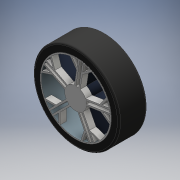
# Autodesk Inventor part: rueda
Saved by Autodesk Inventor 2016 (Build 200138000, 138)
## iProperties
Created: 2017-12-28
Part Number: rueda
Material: Genérico
Document SubType Name: Sheet Metal
Designer: David
Density: 1 g/cm^3
Sheet Metal Rule: Por defecto_mm
Appearance: Valor por defecto
Author: David
Autodesk Inventor part; units mm, degrees
ref_plane "YZ Plane" through (0, 0, 0) normal (1, 0, 0) x (0, 1, 0)
ref_plane "XZ Plane" through (0, 0, 0) normal (0, 1, 0) x (-1, 0, 0)
ref_plane "XY Plane" through (0, 0, 0) normal (0, 0, 1) x (1, 0, 0)
sketch "Boceto1" plane through (0, 0, 0) normal (0, 1, 0) x (-1, 0, 0)
  line L0 (0, 0) -> (10.773409, 0) construction
  line L1 (0, 0) -> (5.876404, 0) construction
  line L2 (0, 0) -> (5.876414, 0) construction
  line L3 (2.696241, -2.108582) -> (2.892291, -2.304632)
  line L4 (2.092671, -2.708608) -> (2.372911, -2.990503)
  line L5 (2.372911, -2.990503) -> (7.29151, -7.938146)
  line L6 (1.666633, -2.989677) -> (4.8298, -6.171522)
  line L7 (4.8298, -6.171522) -> (4.8298, -9.636042)
  line L8 (5.341204, -9.362255) -> (5.341204, -6.665792)
  line L9 (5.341204, -6.665792) -> (6.925478, -8.259421)
  line L10 (2.694469, -2.10681) -> (2.976364, -2.38705)
  line L11 (2.976364, -2.38705) -> (7.924007, -7.305649)
  line L12 (2.975538, -1.680772) -> (6.157383, -4.843939)
  line L13 (6.157383, -4.843939) -> (9.621903, -4.843939)
  line L14 (9.348116, -5.355343) -> (6.651653, -5.355343)
  line L15 (6.651653, -5.355343) -> (8.245282, -6.939617)
  line L16 (7.923737, -7.305381) -> (7.924595, -7.306234)
  line L17 (8.244685, -6.939024) -> (8.246514, -6.940842)
  line L18 (9.347907, -5.355343) -> (9.354174, -5.355343)
  line L19 (9.62164, -4.843939) -> (9.628942, -4.843939)
  line L20 (7.148707, 4.671206) -> (9.1479, 5.697269)
  line L21 (7.98196, 7.235695) -> (7.148707, 4.671206)
  line L22 (6.509596, 4.35916) -> (7.580192, 7.654114)
  line L23 (2.518001, 2.310518) -> (6.509596, 4.35916)
  line L24 (3.189966, 2.093051) -> (9.396738, 5.278608)
  line L25 (3.577407, 1.332656) -> (9.802826, 4.481616)
  line L26 (2.836332, 1.911553) -> (3.189966, 2.093051)
  line L27 (3.222711, 1.153243) -> (3.577407, 1.332656)
  line L28 (3.358369, 0.661201) -> (7.361957, 2.686308)
  line L29 (7.990067, 3.019944) -> (9.995266, 4.03422)
  line L30 (10.554556, 2.186691) -> (7.990067, 3.019944)
  line L31 (7.361957, 2.686308) -> (10.656911, 1.615712)
  line L32 (-2.233509, 8.242307) -> (-2.591569, 10.460723)
  line L33 (-4.414993, 9.827248) -> (-2.233509, 8.242307)
  line L34 (-2.134232, 7.538048) -> (-4.937087, 9.574442)
  line L35 (-1.419328, 3.10875) -> (-2.134232, 7.538048)
  line L36 (-1.004856, 3.680627) -> (-2.116503, 10.568008)
  line L37 (-0.161952, 3.81413) -> (-1.233031, 10.707937)
  line L38 (-0.94152, 3.288215) -> (-1.004856, 3.680627)
  line L39 (-0.100927, 3.421351) -> (-0.161952, 3.81413)
  line L40 (0.408954, 3.398321) -> (-0.279861, 7.831752)
  line L41 (-0.403071, 8.53222) -> (-0.748064, 10.752705)
  line L42 (1.181871, 10.713704) -> (-0.403071, 8.53222)
  line L43 (-0.279861, 7.831752) -> (1.756533, 10.634607)
  line L44 (-8.529092, 0.42282) -> (-10.749577, 0.767813)
  line L45 (-10.710576, -1.162121) -> (-8.529092, 0.42282)
  line L46 (-7.828624, 0.29961) -> (-10.631479, -1.736783)
  line L47 (-3.395193, -0.389204) -> (-7.828624, 0.29961)
  line L48 (-3.811002, 0.181701) -> (-10.704809, 1.25278)
  line L49 (-3.677499, 1.024606) -> (-10.56488, 2.136253)
  line L50 (-3.418223, 0.120676) -> (-3.811002, 0.181701)
  line L51 (-3.285087, 0.961269) -> (-3.677499, 1.024606)
  line L52 (-3.105622, 1.439077) -> (-7.53492, 2.153981)
  line L53 (-8.239179, 2.253258) -> (-10.457595, 2.611318)
  line L54 (-9.82412, 4.434742) -> (-8.239179, 2.253258)
  line L55 (-7.53492, 2.153981) -> (-9.571314, 4.956836)
  line L56 (-3.03776, -7.98099) -> (-4.052036, -9.986188)
  line L57 (-2.204507, -10.545478) -> (-3.03776, -7.98099)
  line L58 (-2.704124, -7.352879) -> (-1.633529, -10.647833)
  line L59 (-0.679017, -3.349292) -> (-2.704124, -7.352879)
  line L60 (-1.350472, -3.568329) -> (-4.499432, -9.793748)
  line L61 (-2.110867, -3.180889) -> (-5.296425, -9.38766)
  line L62 (-1.171059, -3.213633) -> (-1.350472, -3.568329)
  line L63 (-1.929369, -2.827255) -> (-2.110867, -3.180889)
  line L64 (-2.328334, -2.508923) -> (-4.376976, -6.500518)
  line L65 (-4.689022, -7.13963) -> (-5.715085, -9.138822)
  line L66 (-7.253511, -7.972883) -> (-4.689022, -7.13963)
  line L67 (-4.376976, -6.500518) -> (-7.67193, -7.571114)
  arc A0 (3.222711, 1.153243) -> (2.83856, 1.912696) centre (0, 0) ccw
  arc A1 (2.979517, -1.684728) -> (3.358369, 0.661201) centre (0, 0) ccw
  arc A2 (2.092671, -2.708608) -> (2.696245, -2.108576) centre (0, 0) ccw
  arc A3 (-0.68155, -3.354299) -> (1.666633, -2.989677) centre (0, 0) ccw
  arc A4 (2.522993, 2.31308) -> (0.408954, 3.398321) centre (0, 0) ccw
  arc A5 (-0.100927, 3.421351) -> (-0.941919, 3.290687) centre (0, 0) ccw
  arc A6 (-1.420222, 3.11429) -> (-3.105622, 1.439077) centre (0, 0) ccw
  arc A7 (-3.285087, 0.961269) -> (-3.420698, 0.12106) centre (0, 0) ccw
  arc A8 (-3.400738, -0.388343) -> (-2.328334, -2.508923) centre (0, 0) ccw
  arc A9 (-1.929369, -2.827255) -> (-1.172189, -3.215868) centre (0, 0) ccw
  line L68 (-2.205227, -10.543261) -> (-2.202798, -10.551206)
  line L69 (-1.634443, -10.645018) -> (-1.631353, -10.654528)
  line L70 (-4.051656, -9.985437) -> (-4.05282, -9.987739)
  line L71 (-4.499261, -9.793408) -> (-4.499807, -9.794489)
  line L72 (-10.619132, -1.727812) -> (-10.637174, -1.740921)
  line L73 (-10.708499, -1.160612) -> (-10.715477, -1.165682)
  line L74 (-10.747959, 0.767562) -> (-10.751294, 0.76808)
  line L75 (-10.702047, 1.252351) -> (-10.705629, 1.252907)
  line L76 (-4.936194, 9.573793) -> (-4.942782, 9.578579)
  line L77 (-4.413036, 9.825826) -> (-4.419894, 9.830809)
  line L78 (-2.591187, 10.458357) -> (-2.591845, 10.462438)
  line L79 (-2.116332, 10.56695) -> (-2.116636, 10.568828)
  line L80 (7.5795, 7.651986) -> (7.582367, 7.660809)
  line L81 (7.981253, 7.233517) -> (7.983833, 7.241456)
  line L82 (9.145324, 5.695947) -> (9.149446, 5.698063)
  line L83 (9.394975, 5.277704) -> (9.397476, 5.278988)
  circle A10 centre (0, 0) radius 11.15
  arc A11 (9.149446, 5.698063) -> (7.983833, 7.241456) centre (0, 0) ccw
  arc A12 (9.802826, 4.481616) -> (9.397476, 5.278988) centre (0, 0) ccw
  arc A13 (10.554556, 2.186691) -> (9.995266, 4.03422) centre (0, 0) ccw
  arc A14 (9.628942, -4.843939) -> (10.656911, 1.615712) centre (0, 0) ccw
  arc A15 (8.246514, -6.940842) -> (9.354174, -5.355343) centre (0, 0) ccw
  arc A16 (7.29151, -7.938146) -> (7.924595, -7.306234) centre (0, 0) ccw
  arc A17 (5.341204, -9.362255) -> (6.925478, -8.259421) centre (0, 0) ccw
  arc A18 (-5.296425, -9.38766) -> (-4.499807, -9.794489) centre (0, 0) ccw
  arc A19 (-4.05282, -9.987739) -> (-2.202798, -10.551206) centre (0, 0) ccw
  arc A20 (-1.631353, -10.654528) -> (4.8298, -9.636042) centre (0, 0) ccw
  arc A21 (-7.253511, -7.972883) -> (-5.715085, -9.138822) centre (0, 0) ccw
  arc A22 (7.582367, 7.660809) -> (1.756533, 10.634607) centre (0, 0) ccw
  arc A23 (1.181871, 10.713704) -> (-0.748064, 10.752705) centre (0, 0) ccw
  arc A24 (-1.233031, 10.707937) -> (-2.116636, 10.568828) centre (0, 0) ccw
  arc A25 (-2.591845, 10.462438) -> (-4.419894, 9.830809) centre (0, 0) ccw
  arc A26 (-4.942782, 9.578579) -> (-9.571314, 4.956836) centre (0, 0) ccw
  arc A27 (-9.82412, 4.434742) -> (-10.457595, 2.611318) centre (0, 0) ccw
  arc A28 (-10.56488, 2.136253) -> (-10.705629, 1.252907) centre (0, 0) ccw
  arc A29 (-10.751294, 0.76808) -> (-10.715477, -1.165682) centre (0, 0) ccw
  arc A30 (-10.637174, -1.740921) -> (-7.67193, -7.571114) centre (0, 0) ccw
  point P0 (9.147151, 5.696885)
  point P1 (7.981896, 7.235496)
  point P2 (7.58011, 7.653864)
  point P3 (9.396399, 5.278435)
  point P4 (-2.591434, 10.459892)
  point P5 (-4.414824, 9.827125)
  point P6 (-4.936874, 9.574287)
  point P7 (-2.116443, 10.567633)
  point P8 (-10.748746, 0.767684)
  point P9 (-10.710407, -1.161998)
  point P10 (-10.631266, -1.736629)
  point P11 (-10.704433, 1.252722)
  point P12 (-2.204572, -10.54528)
  point P13 (-1.63361, -10.647583)
  dimension "d18" = 360
  constraints: 168 end point, 61 point on circle, 55 point on line, 31 centre point, 5 horizontal, 3 coincident, 2 parallel, 2 vertical, 1 collinear, 171 other
extrude "Extrusión1" add sketch "Boceto1" along normal blind 2
sketch "Boceto7" plane through (0, 2, 0) normal (0, 1, 0) x (1, 0, 0)
  circle A0 centre (0, 0) radius 11.15
  circle A1 centre (0, 0) radius 13.5
  dimension "d31" = 27
  constraints: 2 centre point, 2 coincident
  measures "d31" diameter of A1
extrude "Extrusión5" add sketch "Boceto7" along normal blind 7
sketch "Boceto8" plane through (0, 2, 0) normal (0, -1, 0) x (1, 0, 0)
  circle A0 centre (0, 0) radius 11.15
  circle A1 centre (0, 0) radius 13.5
  dimension "d34" = 27
  constraints: 2 centre point, 2 coincident
  measures "d34" diameter of A1
extrude "Extrusión6" add sketch "Boceto8" along normal blind 1.9
sketch "Boceto9" plane through (0, 2, 0) normal (0, 1, 0) x (1, 0, 0)
  line L0 (3.420698, -0.12106) -> (10.705629, -1.252907)
  line L1 (0.236076, -0.027629) -> (10.705629, -1.252907)
  line L2 (10.705629, -1.252907) -> (10.748719, -0.975566)
  line L3 (10.748719, -0.975566) -> (0.123114, 0.267976)
  line L4 (4.499807, 9.794489) -> (1.172189, 3.215868)
  arc A0 (4.05282, 9.987739) -> (2.202798, 10.551206) centre (0, 0) ccw
  line L5 (4.499807, 9.794489) -> (0.123114, 0.267976)
  line L6 (4.499807, 9.794489) -> (4.281466, 9.891882)
  line L7 (4.281466, 9.891882) -> (-0.176715, 0.162926)
  line L8 (-7.924595, 7.306234) -> (-2.696241, 2.108582)
  line L9 (-0.176715, 0.162926) -> (-7.924595, 7.306234)
  arc A1 (-7.29151, 7.938146) -> (-7.924595, 7.306234) centre (0, 0) ccw
  line L10 (-7.924595, 7.306234) -> (-8.06896, 7.149652)
  line L11 (-8.06896, 7.149652) -> (-0.651971, 0.076302)
  line L12 (-2.83856, -1.912696) -> (-9.397476, -5.278988)
  line L13 (-0.359943, -0.202196) -> (-9.397476, -5.278988)
  line L14 (-9.397476, -5.278988) -> (-9.286303, -5.472188)
  line L15 (-9.286303, -5.472188) -> (0, -0.289682)
  line L16 (0.941919, -3.290687) -> (2.116636, -10.568828)
  line L17 (0.050787, -0.253592) -> (2.116636, -10.568828)
  line L18 (2.116636, -10.568828) -> (2.339959, -10.532783)
  line L19 (2.339959, -10.532783) -> (0.236076, -0.027629)
  line L20 (-0.651971, 0.076302) -> (-0.359943, -0.202196)
  line L21 (0, -0.289682) -> (0.050787, -0.253592)
  constraints: 34 end point, 2 parallel, 2 perpendicular, 1 tangent
extrude "Extrusión7" add sketch "Boceto9" along normal blind 6.5
sketch "Boceto10" plane through (0, 8.5, 0) normal (0, 1, 0) x (1, 0, 0)
  circle A0 centre (0, 0) radius 2.5
  dimension "d39" = 5
  constraints: 1 centre point, 1 coincident
  measures "d39" diameter of A0
extrude "Extrusión8" add sketch "Boceto10" against normal blind 6.5
fillet "Empalme1" radius 0.5 1 edges at (-13.5, 0.1, 0)
fillet "Empalme2" radius 0.5 1 edges at (-13.5, 9, 0)
sketch "Boceto11" plane through (0, 2, 0) normal (0, 1, 0) x (1, 0, 0)
  circle A0 centre (0, 0) radius 11.15
  circle A1 centre (0, 0) radius 10.778695
  point P0 (4.499807, 9.794489)
  constraints: 2 coincident, 1 centre point, 3 other
extrude "Extrusión9" add sketch "Boceto11" along normal blind 6.5
equation "\"Radio_pliegue\" = Grosor"
equation "\"Anchura_desahogo_plegado\" = Grosor"
equation "\"Profundidad_desahogo_plegado\" = 0.5 * Grosor"
equation "\"Tamaño_destalonado\" = 4 * Grosor"
equation "\"Remanente_mínimo\" = 2 * Grosor"
equation "\"Radiodetransición\" = Radio_pliegue"
equation "\"Tamaño_de_radio_de_Jacobi\" = Radio_pliegue"
equation "\"TamañoSeparación\" = Grosor"
equation "\"Grosor\" = 0.5"
